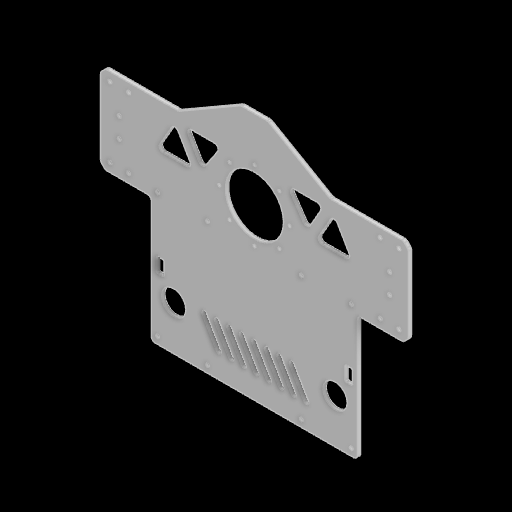
# Autodesk Inventor part: Root
Saved by Autodesk Inventor 2025.2 (Build 292293000, 293)
## iProperties
Created: 2020-05-07
Part Number: Root
Material: Generic
Document SubType Name: Sheet Metal
Designer: valer
Density: 1 g/cm^3
Sheet Metal Rule: Default
Appearance: Default
Author: valer
Autodesk Inventor part; units mm, degrees
ref_plane "YZ Plane" through (0, 0, 0) normal (1, 0, 0) x (0, 1, 0)
ref_plane "XZ Plane" through (0, 0, 0) normal (0, 1, 0) x (-1, 0, 0)
ref_plane "XY Plane" through (0, 0, 0) normal (0, 0, 1) x (1, 0, 0)
sketch "Base" plane through (0, 0, 0) normal (0, 0, 1) x (1, 0, 0)
  circle A0 centre (-56.25, 0) radius 2.75 construction
  circle A1 centre (0, -56.25) radius 2.75 construction
  circle A2 centre (0, 56.25) radius 2.75 construction
  circle A3 centre (39.7748, -39.7748) radius 2.75 construction
  circle A4 centre (-39.7748, 39.7748) radius 2.75 construction
  circle A5 centre (-39.7748, -39.7748) radius 2.75 construction
  circle A6 centre (39.7748, 39.7748) radius 2.75 construction
  circle A7 centre (56.25, 0) radius 2.75 construction
  circle A8 centre (0, 0) radius 45 construction
  circle A9 centre (0, 0) radius 61
  line L0 (0, -352) -> (0, 222) construction
  line L1 (-344.741, 0) -> (344.741, 0) construction
  circle A10 centre (0, 0) radius 46.5
  circle A11 centre (-56.25, 0) radius 2.25
  circle A12 centre (-39.7748, -39.7748) radius 2.25
  circle A13 centre (0, -56.25) radius 2.25
  circle A14 centre (39.7748, -39.7748) radius 2.25
  circle A15 centre (56.25, 0) radius 2.25
  circle A16 centre (39.7748, 39.7748) radius 2.25
  circle A17 centre (0, 56.25) radius 2.25
  circle A18 centre (-39.7748, 39.7748) radius 2.25
  line L2 (-121.2436, 70) -> (0, 140)
  line L3 (0, 140) -> (121.2436, 70)
  line L4 (121.2436, 70) -> (121.2436, -70)
  line L5 (121.2436, -70) -> (0, -140)
  line L6 (0, -140) -> (-121.2436, -70)
  line L7 (-121.2436, -70) -> (-121.2436, 70)
  line L8 (121.2436, 70) -> (246.2436, 70)
  line L9 (246.2436, 70) -> (246.2436, -70)
  line L10 (246.2436, -70) -> (121.2436, -70)
  line L11 (-121.2436, 70) -> (-246.2436, 70)
  line L12 (-246.2436, 70) -> (-246.2436, -70)
  line L13 (-246.2436, -70) -> (-121.2436, -70)
  line L14 (165, -70) -> (165, -270)
  line L15 (165, -270) -> (0, -270)
  line L16 (-165, -70) -> (-165, -270)
  line L17 (-165, -270) -> (0, -270)
  point P0 (0, 0)
  dimension "d91" = 1.5
  dimension "d92" = 4.5
  dimension "d164" = 125
  dimension "d165" = 140
  dimension "d173" = 165
  dimension "d174" = 200
  measures "d91" radial gap between concentric circles of A10 A8
  measures "d92" diameter of A11
  measures "d164" distance of L3.end L8.end
  measures "d165" distance of L8.end L9.end
  measures "d173" distance of L14.end L15.end
  measures "d174" distance between parallel lines of L10 L15
extrude "Plate1" add sketch "Base" against normal blind 5 contours A9 | L2 L3 L4 L5 L6 L7 | L7 L13 L12 L11 | L6 L5 L10 L14 L15 L17 L16 L13 | L8 L9 L10 L4
sketch "LegMountHoles" plane through (0, 0, -5) normal (0, 0, -1) x (-1, 0, 0)
  line L0 (-216.2436, 44.9096) -> (-216.2436, -35.0904) construction
  line L1 (-201.2436, 56) -> (-231.2436, 56) construction
  circle A0 centre (-201.2436, 56) radius 3
  circle A1 centre (-231.2436, 56) radius 3
  circle A2 centre (-216.2436, 16) radius 3
  line L2 (344.741, 0) -> (-344.741, 0) construction
  line L3 (0, -352) -> (0, 222) construction
  circle A3 centre (201.2436, 56) radius 3
  circle A4 centre (231.2436, 56) radius 3
  circle A5 centre (216.2436, 16) radius 3
  circle A6 centre (-201.2436, -56) radius 3
  circle A7 centre (-231.2436, -56) radius 3
  circle A8 centre (-216.2436, -16) radius 3
  circle A9 centre (201.2436, -56) radius 3
  circle A10 centre (231.2436, -56) radius 3
  circle A11 centre (216.2436, -16) radius 3
  line L4 (-246.2436, -70) -> (-246.2436, 70) projected
  point P0 (0, 0)
  point P1 (-216.2436, 56)
  dimension "d93" = 6
  dimension "d94" = 30
  dimension "d95" = 40
  dimension "d161" = 16
  dimension "d166" = 30
  constraints: 12 centre point, 9 symmetric about line, 4 end point, 2 coincident, 2 equal radius, 2 point on line, 1 horizontal, 1 midpoint, 1 perpendicular, 9 other
  measures "d93" diameter of A0
  measures "d94" distance of L1.start L1.end
  measures "d95" distance from line of L1 A2.centre
  measures "d161" distance from line of L2 A2.centre
  measures "d166" distance between parallel lines of L4 L0
extrude "LegMountHolesFeature" cut sketch "LegMountHoles" against normal blind 5
chamfer "FrontChamferFeature" distance 25 angle 45 1 edges at (0, 140, -2.5)
chamfer "SideChamfersFeature" distance 8 angle 45 4 edges at (246.2436, 70, -2.5) (246.2436, -70, -2.5) (-246.2436, 70, -2.5) (-246.2436, -70, -2.5)
fillet "FilletsFeature" radius 6 16 edges at (165, -270, -2.5) (-165, -270, -2.5) (-238.2436, -70, -2.5) (-246.2436, -62, -2.5) (-165, -70, -2.5) (165, -70, -2.5) (238.2436, -70, -2.5) (246.2436, -62, -2.5) (246.2436, 62, -2.5) (238.2436, 70, -2.5) (121.2436, 70, -2.5) (21.6506, 127.5, -2.5) (-21.6506, 127.5, -2.5) (-121.2436, 70, -2.5) (-238.2436, 70, -2.5) (-246.2436, 62, -2.5)
sketch "BatteryContactHoles" plane through (0, 0, -5) normal (0, 0, -1) x (-1, 0, 0)
  circle A0 centre (-129.1, -199.15) radius 18.4 construction
  circle A1 centre (129.1, -199.15) radius 18.4 construction
  circle A2 centre (129.1, -199.15) radius 19.4
  circle A3 centre (-129.1, -199.15) radius 19.4
  point P0 (0, 0)
  dimension "d199" = 1
  constraints: 2 centre point, 2 coincident, 1 equal radius
  measures "d199" radial gap between concentric circles of A2 A1
extrude "BatteryContactHolesFeature" cut sketch "BatteryContactHoles" against normal blind 5
sketch "BatteryMountHoles" plane through (0, 0, -5) normal (0, 0, -1) x (-1, 0, 0)
  circle A0 centre (-155, -259) radius 3 projected
  circle A1 centre (-75, -259) radius 3 projected
  circle A2 centre (75, -259) radius 3 projected
  circle A3 centre (155, -259) radius 3 projected
  circle A4 centre (-155, -59.5) radius 3 projected
  circle A5 centre (-75, -59.5) radius 3 projected
  circle A6 centre (75, -59.5) radius 3 projected
  circle A7 centre (155, -59.5) radius 3 projected
  point P0 (0, 0)
extrude "BatteryMountHolesFeature" cut sketch "BatteryMountHoles" against normal blind 5
sketch "BatteryStrapHoles" plane through (0, 0, -5) normal (0, 0, -1) x (-1, 0, 0)
  line L0 (-156.75, -148) -> (-144.75, -148)
  line L1 (-144.75, -148) -> (-144.75, -171.5)
  line L2 (-144.75, -171.5) -> (-156.75, -171.5)
  line L3 (-156.75, -171.5) -> (-156.75, -148)
  line L4 (0, -349.5) -> (0, 207) construction
  line L5 (-156.75, -148) -> (-152.25, -148) projected
  line L6 (-152.25, -171.5) -> (-156.75, -171.5) projected
  line L7 (156.75, -148) -> (144.75, -148)
  line L8 (144.75, -148) -> (144.75, -171.5)
  line L9 (144.75, -171.5) -> (156.75, -171.5)
  line L10 (156.75, -171.5) -> (156.75, -148)
  point P0 (0, 0)
  dimension "d204" = 12
  constraints: 16 end point, 4 symmetric about line, 2 parallel, 1 horizontal, 1 perpendicular
  measures "d204" distance of L0.start L0.end
extrude "BatteryStrapHolesFeature" cut sketch "BatteryStrapHoles" against normal blind 5
fillet "BatteryStrapHoleFilletsFeature" radius 2 8 edges at (156.75, -148, -2.5) (144.75, -148, -2.5) (156.75, -171.5, -2.5) (144.75, -171.5, -2.5) (-144.75, -148, -2.5) (-156.75, -148, -2.5) (-156.75, -171.5, -2.5) (-144.75, -171.5, -2.5)
sketch "BaseCuts" plane through (0, 0, -5) normal (0, 0, -1) x (-1, 0, 0)
  line L0 (-110.9284, 54.5665) -> (-83.9364, 7.815)
  line L1 (-83.9364, 7.815) -> (-52.7204, 54.5665)
  line L2 (-52.7204, 54.5665) -> (-110.9284, 54.5665)
  line L3 (-97.8781, 0) -> (-127.3375, 51.0252)
  line L4 (-127.3375, 51.0252) -> (-156.7969, 0)
  line L5 (-156.7969, 0) -> (-97.8781, 0)
  line L6 (0, -349.5) -> (0, 207) construction
  line L7 (110.9284, 54.5665) -> (83.9364, 7.815)
  line L8 (83.9364, 7.815) -> (52.7204, 54.5665)
  line L9 (52.7204, 54.5665) -> (110.9284, 54.5665)
  line L10 (97.8781, 0) -> (127.3375, 51.0252)
  line L11 (127.3375, 51.0252) -> (156.7969, 0)
  line L12 (156.7969, 0) -> (97.8781, 0)
  line L13 (344.741, 0) -> (-344.741, 0) construction
  point P0 (0, 0)
  dimension "d218" = 60
  dimension "d219" = 60
  constraints: 24 end point, 6 symmetric about line, 2 horizontal, 1 collinear, 1 parallel
  measures "d218" angle of L5 L3
  measures "d219" angle of L4 L5
extrude "BaseCutsFeature" cut sketch "BaseCuts" against normal blind 5
fillet "BaseCutFilletsFeature" radius 6 12 edges at (52.7204, 54.5665, -2.5) (110.9284, 54.5665, -2.5) (83.9364, 7.815, -2.5) (127.3375, 51.0252, -2.5) (156.7969, 0, -2.5) (97.8781, 0, -2.5) (-110.9284, 54.5665, -2.5) (-52.7204, 54.5665, -2.5) (-83.9364, 7.815, -2.5) (-97.8781, 0, -2.5) (-127.3375, 51.0252, -2.5) (-156.7969, 0, -2.5)
sketch "BackVents" plane through (0, 0, -5) normal (0, 0, -1) x (-1, 0, 0)
  line L0 (-83, -230) -> (-59.906, -190) construction
  line L1 (-86.4641, -228) -> (-63.3701, -188)
  line L2 (-56.4419, -192) -> (-79.5359, -232)
  arc A0 (-86.4641, -228) -> (-79.5359, -232) centre (-83, -230) ccw
  arc A1 (-56.4419, -192) -> (-63.3701, -188) centre (-59.906, -190) ccw
  line L3 (344.741, 0) -> (-344.741, 0) construction
  line L4 (0, -349.5) -> (0, 207) construction
  line L5 (159, -270) -> (-159, -270) projected
  line L6 (-83, -230) -> (165, -230) construction
  line L7 (-59.906, -190) -> (165, -190) construction
  line L8 (-165, -264) -> (-165, -76) projected
  line L9 (165, -76) -> (165, -264) projected
  arc A2 (-36.4419, -192) -> (-43.3701, -188) centre (-39.906, -190) ccw
  line L10 (-66.4641, -228) -> (-43.3701, -188)
  line L11 (-36.4419, -192) -> (-59.5359, -232)
  arc A3 (-66.4641, -228) -> (-59.5359, -232) centre (-63, -230) ccw
  arc A4 (-16.4419, -192) -> (-23.3701, -188) centre (-19.906, -190) ccw
  line L12 (-46.4641, -228) -> (-23.3701, -188)
  line L13 (-16.4419, -192) -> (-39.5359, -232)
  arc A5 (-46.4641, -228) -> (-39.5359, -232) centre (-43, -230) ccw
  arc A6 (3.5581, -192) -> (-3.3701, -188) centre (0.094, -190) ccw
  line L14 (-26.4641, -228) -> (-3.3701, -188)
  line L15 (3.5581, -192) -> (-19.5359, -232)
  arc A7 (-26.4641, -228) -> (-19.5359, -232) centre (-23, -230) ccw
  arc A8 (23.5581, -192) -> (16.6299, -188) centre (20.094, -190) ccw
  line L16 (-6.4641, -228) -> (16.6299, -188)
  line L17 (23.5581, -192) -> (0.4641, -232)
  arc A9 (-6.4641, -228) -> (0.4641, -232) centre (-3, -230) ccw
  arc A10 (43.5581, -192) -> (36.6299, -188) centre (40.094, -190) ccw
  line L18 (13.5359, -228) -> (36.6299, -188)
  line L19 (43.5581, -192) -> (20.4641, -232)
  arc A11 (13.5359, -228) -> (20.4641, -232) centre (17, -230) ccw
  arc A12 (63.5581, -192) -> (56.6299, -188) centre (60.094, -190) ccw
  line L20 (33.5359, -228) -> (56.6299, -188)
  line L21 (63.5581, -192) -> (40.4641, -232)
  arc A13 (33.5359, -228) -> (40.4641, -232) centre (37, -230) ccw
  arc A14 (83.5581, -192) -> (76.6299, -188) centre (80.094, -190) ccw
  line L22 (53.5359, -228) -> (76.6299, -188)
  line L23 (83.5581, -192) -> (60.4641, -232)
  arc A15 (53.5359, -228) -> (60.4641, -232) centre (57, -230) ccw
  point P0 (0, 0)
  point P1 (-71.453, -210)
  dimension "d223" = 4
  dimension "d224" = 40
  dimension "d225" = 80
  dimension "d226" = 60
  dimension "d227" = 82
  dimension "d230" = 20
  constraints: 40 end point, 32 point on circle, 16 centre point, 4 tangent, 3 horizontal, 2 point on line, 1 midpoint, 1 parallel, 70 other
  measures "d223" radius of A1
  measures "d224" distance from line of L5 L0.start
  measures "d225" distance from line of L5 L0.end
  measures "d226" angle of L0 L6
  measures "d227" distance from line of L8 L0.start
  measures "d230" distance of L0.end A2.centre
extrude "VentsFeature" cut sketch "BackVents" against normal blind 5
equation "\"d97\" = Thickness"
equation "\"d33\" = Thickness"
equation "\"BendRadius\" = Thickness"
equation "\"BendReliefWidth\" = Thickness"
equation "\"BendReliefDepth\" = 0.5 * Thickness"
equation "\"TransitionRadius\" = BendRadius"
equation "\"JacobiRadiusSize\" = BendRadius"
equation "\"GapSize\" = Thickness"
equation "\"Thickness\" = 5"
body "Solid1"
